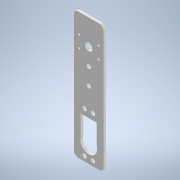
# Autodesk Inventor part: 3
Saved by Autodesk Inventor 2021 (Build 250183000, 183)
## iProperties
Created: 2021-03-30
Part Number: 3
Material: Genérico
Document SubType Name: Modeling
Designer: diego
Density: 1 g/cm^3
Appearance: Valor por defecto
Author: diego
Autodesk Inventor part; units mm, degrees
ref_plane "YZ Plane" through (0, 0, 0) normal (1, 0, 0) x (0, 1, 0)
ref_plane "XZ Plane" through (0, 0, 0) normal (0, 1, 0) x (-1, 0, 0)
ref_plane "XY Plane" through (0, 0, 0) normal (0, 0, 1) x (1, 0, 0)
sketch "Boceto1" plane through (0, 0, 0) normal (0, 0, 1) x (1, 0, 0)
  line L0 (0, 5) -> (0, 145)
  line L1 (5, 150) -> (30, 150)
  line L2 (35, 145) -> (35, 5)
  line L3 (30, 0) -> (5, 0)
  arc A0 (5, 150) -> (0, 145) centre (5, 145) ccw
  arc A1 (35, 145) -> (30, 150) centre (30, 145) ccw
  arc A2 (0, 5) -> (5, 0) centre (5, 5) ccw
  arc A3 (30, 0) -> (35, 5) centre (30, 5) ccw
  circle A4 centre (17.5, 120) radius 4.5
  circle A5 centre (17.5, 100) radius 2.5
  circle A6 centre (17.5, 80) radius 2.5
  circle A7 centre (17.5, 20) radius 6.5
  circle A8 centre (22.5, 54.5) radius 2.5
  circle A9 centre (12.5, 54.5) radius 2.5
  circle A10 centre (12.5, 6) radius 2.5
  circle A11 centre (22.5, 6) radius 2.5
  circle A12 centre (6, 127) radius 1.25
  circle A13 centre (6, 113) radius 1.25
  circle A14 centre (29, 113) radius 1.25
  circle A15 centre (29, 127) radius 1.25
  point P0 (0, 0)
  constraints: 16 centre point, 8 end point, 8 point on circle, 8 tangent, 3 equal radius, 3 perpendicular, 2 point on line, 1 vertical
extrude "Extrusión1" add sketch "Boceto1" along normal blind 3
sketch "Boceto2" plane through (0, 0, 0) normal (0, 0, -1) x (-1, 0, 0)
  circle A0 centre (-17.5, 20) radius 6.5 projected
  arc A1 (-27, 23.1225) -> (-8, 23.1225) centre (-17.5, 20) ccw
  line L0 (-17.5, 47) -> (-27, 47)
  line L1 (-27, 47) -> (-8, 47)
  line L2 (-8, 47) -> (-8, 23.1225)
  line L3 (-27, 47) -> (-27, 23.1225)
  point P0 (0, 0)
  constraints: 8 end point, 2 point on circle, 1 centre point, 1 coincident, 1 perpendicular, 1 point on line
extrude "Extrusión2" cut sketch "Boceto2" against normal blind 10
